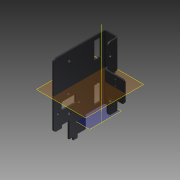
# Autodesk Inventor part: D-003
Saved by Autodesk Inventor 2015 (Build 190159000, 159)
## iProperties
Created: 2014-01-21
Part Number: D-003
Material: Steel
Document SubType Name: Chapa
Designer: O.Martin
Mass: 157.649 g
Surface Area: 219.047 cm^2
Volume: 20.0827 cm^3
Density: 7.85 g/cm^3
Project: WITBOXprinter_K01
Description: PLACA LATERAL MOTOR
Stock Number: 2014000004
Sheet Metal Rule: Por defecto
Appearance: Rubber - Black - Version 1.1
GlobalPropertyList: <PropertyList/>
Company: MARCHA TECHNOLOGY
Author: O.Martin
Autodesk Inventor part; units mm, degrees
ref_plane "YZ Plane" through (0, 0, 0) normal (1, 0, 0) x (0, 1, 0)
ref_plane "XZ Plane" through (0, 0, 0) normal (0, 1, 0) x (-1, 0, 0)
sketch "Boceto1" plane through (0, 0, 0) normal (0, 0, 1) x (1, 0, 0)
  line L0 (0, -25) -> (0, 25) construction
  circle A0 centre (0, 25) radius 4 construction
  circle A1 centre (0, 25) radius 7.5 construction
  line L1 (-7.5399, -37.5) -> (-7.5399, 37.5)
  line L2 (-7.5399, 37.5) -> (12.4601, 37.5)
  line L3 (12.4601, 37.5) -> (12.4601, 22)
  line L4 (12.4601, 22) -> (10.4601, 22)
  line L5 (10.4601, 22) -> (10.4601, 35.5)
  line L6 (10.4601, 35.5) -> (-5.5399, 35.5)
  line L7 (-5.5399, 35.5) -> (-5.5399, -35.5)
  line L8 (-5.5399, -35.5) -> (40.4601, -35.5)
  line L9 (40.4601, -35.5) -> (40.4601, -5)
  line L10 (40.4601, -5) -> (42.4601, -5)
  line L11 (42.4601, -5) -> (42.4601, -37.5)
  line L12 (42.4601, -37.5) -> (-7.5399, -37.5)
  line L13 (-5.5399, 19.9443) -> (-7.5399, 19.9443) construction
  line L14 (-5.5399, 30.0557) -> (-7.5399, 30.0557) construction
  line L15 (-5.5399, -35.5) -> (-5.5399, -37.5)
  point P0 (-7.5399, 0)
  point P1 (0, 0)
  point P2 (0, 0)
  dimension "d4" = 2
  dimension "d5" = 2
  dimension "d6" = 2
  dimension "d7" = 2
  dimension "d46" = 12.5
  dimension "d47" = 75
  dimension "d49" = 3
  dimension "d87" = 15
  dimension "d88" = 20
  dimension "d89" = 8
  dimension "d93" = 32.5
  dimension "d94" = 50
  dimension "d198" = 10.1114
  constraints: 32 end point, 12 parallel, 5 point on line, 4 perpendicular, 3 coincident, 2 centre point, 2 midpoint, 2 point on circle, 1 horizontal alignment, 1 vertical
  measures "d4" distance between parallel lines of L1 L7
  measures "d5" distance of L9.end L10.end
  measures "d6" distance between parallel lines of L12 L8
  measures "d7" distance between parallel lines of L2 L6
  measures "d46" distance from line of L2 L0.end
  measures "d47" distance between parallel lines of L12 L2
  measures "d49" distance from line of A0.centre L4
  measures "d87" diameter of A1
  measures "d88" distance of L1.end L2.end
  measures "d89" diameter of A0
  measures "d93" distance of L10.end L11.end
  measures "d94" distance of L11.end L1.start
  measures "d198" distance between parallel lines of L13 L14
extrude "Extrusión1" add sketch "Boceto1" along normal mid plane 90 contours L1 L2 L3 L4 L5 L6 L7 L15 L12
fillet "Empalme1" radius 4 6 edges at (-7.5399, 37.5, 0) (12.4601, 37.5, 0) (11.4601, 22, 45) (11.4601, 22, -45) (-6.5399, -37.5, 45) (-6.5399, -37.5, -45)
fillet "Empalme1" radius 2 2 edges at (-5.5399, 35.5, 0) (10.4601, 35.5, 0)
sketch "Boceto2" plane through (-7.5399, -33.5, 45) normal (-1, 0, 0) x (0, 0, 1)
  line L0 (-84.6, 63.3744) -> (-60.4, 63.3744)
  line L1 (-60.4, 63.3744) -> (-60.4, 53.6256)
  line L2 (-60.4, 53.6256) -> (-84.6, 53.6256)
  line L3 (-84.6, 53.6256) -> (-84.6, 63.3744)
  line L4 (-29.6, 53.6256) -> (-5.4, 53.6256)
  line L5 (-5.4, 53.6256) -> (-5.4, 63.3744)
  line L6 (-5.4, 63.3744) -> (-29.6, 63.3744)
  line L7 (-29.6, 63.3744) -> (-29.6, 53.6256)
  line L8 (-84.6, 18.5) -> (-5.4, 18.5) construction
  line L9 (-5.4, 18.5) -> (-5.4, 58.5) construction
  line L10 (-5.4, 58.5) -> (-84.6, 58.5) construction
  line L11 (-84.6, 58.5) -> (-84.6, 18.5) construction
  line L12 (0, 71) -> (-90, 71) projected
  line L13 (0, 0) -> (0, 67) projected
  line L14 (-72.5, 63.3744) -> (-72.5, 53.6256) construction
  line L15 (-90, 67) -> (0, 67) construction
  line L16 (-17.5, 63.3744) -> (-17.5, 53.6256) construction
  circle A0 centre (-60.4, 58.5) radius 1
  circle A1 centre (-29.6, 58.5) radius 1
  point P0 (-45, 18.5)
  point P1 (-12.5, 18.5)
  point P2 (-77.5, 18.5)
  point P3 (-72.5, 58.5)
  point P4 (-17.5, 58.5)
  point P5 (-45, 58.5)
  point P6 (-45, 67)
  dimension "d33" = 24.2
  dimension "d36" = 65
  dimension "d45" = 40
  dimension "d48" = 9.7488
  dimension "d103" = 12.5
  dimension "d165" = 12.5
  dimension "d186" = 55
  dimension "d286" = 2
  constraints: 28 end point, 11 midpoint, 8 parallel, 6 point on line, 5 perpendicular, 3 horizontal, 3 vertical alignment, 2 centre point, 1 equal radius
  measures "d33" distance of L4.start L4.end
  measures "d36" distance of point (-12.5, 18.5) point (-77.5, 18.5)
  measures "d45" distance between parallel lines of L10 L8
  measures "d48" distance of L4.end L5.end
  measures "d103" distance between parallel lines of L12 L10
  measures "d165" distance from line of L13 point (-12.5, 18.5)
  measures "d186" distance between parallel lines of L16 L14
  measures "d286" diameter of A0
extrude "Extrusión2" cut sketch "Boceto2" against normal blind 5
hole "Agujero2" at (-7.5399, -15, 32.5) at (-7.5399, -15, -32.5) direction (1, 0, 0) diameter 4 end through all
sketch "Boceto5" plane through (-7.5399, -33.5, 45) normal (-1, 0, 0) x (0, 0, 1)
  line L0 (-68.5, 27.2) -> (-57.5, 27.2)
  line L1 (-57.5, 27.2) -> (-57.5, 7.2)
  line L2 (-57.5, 7.2) -> (-68.5, 7.2)
  line L3 (-68.5, 7.2) -> (-68.5, 27.2)
  circle A0 centre (-77.5, 18.5) radius 2 projected
  line L4 (-90, 67) -> (-90, 0) projected
  line L5 (-69.5, 32.2) -> (-69.5, 2.2) construction
  point P0 (-63, 17.2)
  point P1 (-63, 27.2)
  point P2 (-68.5, 17.2)
  point P3 (-69.5, 17.2)
  dimension "d63" = 20
  dimension "d136" = 1.3
  dimension "d200" = 30
  dimension "d257" = 8
  dimension "d293" = 9
  dimension "d294" = 11
  constraints: 10 end point, 3 midpoint, 3 parallel, 2 horizontal alignment, 1 coincident, 1 horizontal, 1 perpendicular, 1 vertical alignment
  measures "d63" distance of L2.end L0.start
  measures "d136" vertical distance of point (-77.5, 18.5) point (-68.5, 17.2)
  measures "d200" distance of L5.start L5.end
  measures "d257" distance from line of A0.centre L5
  measures "d293" distance from line of L3 point (-77.5, 18.5)
  measures "d294" distance of L1.end L2.end
extrude "Extrusión4" cut sketch "Boceto5" against normal blind 3 contours L0 L1 L2 L3
fillet "Empalme3" radius 2 4 edges at (-6.5399, -6.3, -23.5) (-6.5399, -6.3, -12.5) (-6.5399, -26.3, -12.5) (-6.5399, -26.3, -23.5)
hole "Agujero5" at (-7.5399, 25, -27.5) at (-7.5399, 25, 27.5) direction (1, 0, 0) diameter 3.242 end through all thread size "M4x0.7" class "6H" standard "ISO Metric profile"
hole "Agujero6" at (-7.5399, -1.3, -24.5) at (-7.5399, -31.3, -24.5) direction (1, 0, 0) diameter 3.242 depth 8 tip angle 118 thread size "M4x0.7" class "6H" standard "ISO Metric profile"
sketch "Boceto7" plane through (-7.5399, -33.5, 45) normal (-1, 0, 0) x (0, 0, 1)
  circle A0 centre (-77.5, 18.5) radius 2 projected
  circle A1 centre (-12.5, 18.5) radius 2 projected
  line L0 (-90, 67) -> (-90, 0) projected
  line L1 (-12.5, 28.5) -> (-12.5, 8.5) construction
  line L2 (-77.5, 28.5) -> (-77.5, 8.5) construction
  dimension "d113" = 20
  constraints: 6 coincident, 4 end point, 3 parallel, 2 midpoint
  measures "d113" distance of L1.start L1.end
hole "Agujero8" [suppressed]
sketch "Boceto8" plane through (-3.5399, 37.5, -45) normal (0, 1, 0) x (1, 0, 0)
  line L0 (0, -90) -> (12, -90) projected
  line L1 (4.2, -20) -> (4.2, -70) construction
  line L2 (-4, 0) -> (-4, -90) construction
  point P0 (4.2, -45)
  dimension "d121" = 8.2
  dimension "d122" = 50
  dimension "d169" = 20
  constraints: 2 coincident, 2 end point, 1 midpoint, 1 perpendicular
  measures "d121" distance between parallel lines of L2 L1
  measures "d122" distance of L1.start L1.end
  measures "d169" distance from line of L0 point (4.2, -70)
hole "Agujero9" [suppressed]
sketch "Boceto10" plane through (-7.5399, -33.5, 45) normal (-1, 0, 0) x (0, 0, 1)
  line L0 (-4, -4) -> (-86, -4) projected
  line L1 (-90, 67) -> (-90, 0) projected
  line L2 (-90, 18) -> (-86, 18)
  line L3 (-86, 18) -> (-86, 8)
  line L4 (-86, 8) -> (-90, 8)
  line L5 (-90, 8) -> (-90, 18)
  dimension "d137" = 4
  dimension "d139" = 10
  dimension "d195" = 22
  constraints: 8 end point, 2 parallel, 1 horizontal, 1 perpendicular, 1 point on line
  measures "d137" distance between parallel lines of L1 L3
  measures "d139" distance of L2.end L3.end
  measures "d195" distance between parallel lines of L2 L0
extrude "Extrusión6" cut sketch "Boceto10" against normal through all
sketch "Boceto14" plane through (0, 0, 0) normal (0, 0, 1) x (1, 0, 0)
  line L0 (10.4601, 22) -> (12.4601, 22) projected
  line L1 (12.4601, 22) -> (12.4601, 21)
  arc A0 (12.4601, 21) -> (14.4601, 19) centre (14.4601, 21) ccw
  line L2 (14.4601, 19) -> (40.4601, 19)
  line L3 (40.4601, 19) -> (40.4601, 17)
  line L4 (40.4601, 17) -> (14.4601, 17)
  arc A1 (10.4601, 21) -> (14.4601, 17) centre (14.4601, 21) ccw
  line L5 (10.4601, 21) -> (10.4601, 22)
  dimension "d161" = 4
  dimension "d189" = 5
  dimension "d190" = 30
  constraints: 10 end point, 4 point on circle, 4 tangent, 3 parallel, 2 centre point, 2 perpendicular, 1 concentric
  measures "d161" radius of A1
  measures "d189" distance between parallel lines of L0 L4
  measures "d190" distance between parallel lines of L5 L3
extrude "Extrusión8" add sketch "Boceto14" along normal mid plane 30
sketch "Boceto15" plane through (14.4601, 19, 15) normal (0, 1, 0) x (1, 0, 0)
  line L0 (0, 0) -> (26, 0) projected
  line L1 (26, 0) -> (26, 30) projected
  line L2 (0, 0) -> (0, 30) projected
  line L3 (13, 4.5) -> (13, 12.5) construction
  dimension "d170" = 13
  dimension "d171" = 4.5
  dimension "d172" = 8
  constraints: 2 coincident, 2 end point, 1 parallel
  measures "d170" distance between parallel lines of L1 L3
  measures "d171" distance from line of L0 L3.start
  measures "d172" distance of L3.start L3.end
hole "Agujero11" at (27.4601, 19, 10.5) at (27.4601, 19, 2.5) direction (0, -1, 0) diameter 2.459 end through all thread size "M3x0.5" class "6H" standard "ISO Metric profile"
fillet "Empalme4" radius 4 2 edges at (40.4601, 18, 15) (40.4601, 18, -15)
feature "Desplazar cara1" [suppressed]
sketch "Boceto18" plane through (-3.5399, 37.5, -45) normal (0, 1, 0) x (1, 0, 0)
  line L0 (0, -90) -> (0, 0) projected
  line L1 (16, -90) -> (16, 0) projected
  line L2 (16, -42.25) -> (2, -42.25)
  line L3 (2, -42.25) -> (2, -39.75)
  line L4 (2, -39.75) -> (16, -39.75)
  line L5 (16, -39.75) -> (16, -42.25)
  line L6 (16, -47.75) -> (2, -47.75)
  line L7 (2, -47.75) -> (2, -50.25)
  line L8 (2, -50.25) -> (16, -50.25)
  line L9 (16, -50.25) -> (16, -47.75)
  line L10 (2, -42.25) -> (2, -47.75) construction
  line L11 (12, 0) -> (12, -90) projected
  line L12 (16, -42.25) -> (16, -47.75)
  line L13 (11, -42.25) -> (11, -47.75)
  point P0 (2, -45)
  point P1 (0, -45)
  dimension "d202" = 5.5
  dimension "d203" = 2.5
  dimension "d207" = 1
  dimension "d208" = 9
  constraints: 22 end point, 5 parallel, 4 point on line, 3 perpendicular, 2 equal length, 2 horizontal, 2 midpoint, 1 collinear, 1 horizontal alignment
  measures "d202" distance between parallel lines of L6 L2
  measures "d203" distance of L2.end L3.end
  measures "d207" distance between parallel lines of L11 L13
  measures "d208" distance between parallel lines of L3 L13
extrude "Extrusión11" cut sketch "Boceto18" against normal blind 8
fillet "Redondeo de esquina1" radius 1.25 8 edges at (-1.5399, 36.5, -5.25) (-1.5399, 36.5, -2.75) (-1.5399, 36.5, 2.75) (-1.5399, 36.5, 5.25) (7.4601, 36.5, 2.75) (7.4601, 36.5, -2.75) (11.4601, 29.5, -5.25) (11.4601, 29.5, 5.25)
sketch "Boceto21" plane through (12.4601, 26, 45) normal (1, 0, 0) x (0, 0, -1)
  line L0 (49, 3.5) -> (41, 3.5) projected
  line L1 (39.75, 11.5) -> (0, 11.5) projected
  point P0 (45, -1)
  point P1 (45, 3.5)
  dimension "d224" = 12.5
  constraints: 1 midpoint, 1 vertical alignment
  measures "d224" distance from line of point (45, -1) L1
hole "Agujero12" [suppressed]
sketch "Boceto22" plane through (-7.5399, -33.5, 45) normal (-1, 0, 0) x (0, 0, 1)
  line L0 (-90, 67) -> (-90, 0)
  line L1 (-90, 18) -> (-109, 18)
  line L2 (-109, 18) -> (-109, 24)
  line L3 (-109, 24) -> (-113, 24)
  line L4 (-113, 24) -> (-113, 30)
  line L5 (-113, 30) -> (-90, 30)
  line L6 (-90, 67) -> (-90, 18) projected
  dimension "d232" = 12
  dimension "d233" = 6
  dimension "d234" = 19
  dimension "d235" = 4
  constraints: 12 end point, 2 parallel, 2 perpendicular, 2 point on line
  measures "d232" distance between parallel lines of L1 L5
  measures "d233" distance of L3.end L4.end
  measures "d234" distance of L1.start L1.end
  measures "d235" distance of L2.end L3.end
extrude "Extrusión13" add sketch "Boceto22" against normal up to surface (2 mm away)
ref_plane "Plano de trabajo1" through (0, 0, -47) normal (0, 0, -1) x (-1, 0, 0)
sketch "Boceto23" plane through (0, 0, -47) normal (0, 0, -1) x (-1, 0, 0)
  line L0 (5.5399, -3.5) -> (7.5399, -3.5) projected
  line L1 (7.5399, -3.5) -> (7.5399, 6.5)
  arc A0 (9.3655, 8.4924) -> (7.5399, 6.5) centre (9.5399, 6.5) ccw
  line L2 (9.3655, 8.4924) -> (23.3123, 9.7126)
  line L3 (23.3123, 9.7126) -> (23.138, 11.705)
  line L4 (23.138, 11.705) -> (9.1912, 10.4848)
  arc A1 (9.1912, 10.4848) -> (5.5399, 6.5) centre (9.5399, 6.5) ccw
  line L5 (5.5399, -3.5) -> (5.5399, 6.5)
  line L6 (9.3655, 8.4924) -> (306.3655, 8.4924) construction
  line L7 (23.3123, 9.7126) -> (306.3655, 34.4765) construction
  line L8 (306.3655, 8.4924) -> (306.3655, 34.4765) construction
  dimension "d239" = 2
  dimension "d287" = 10
  dimension "d288" = 14
  dimension "d289" = 95
  dimension "d290" = 2
  dimension "d291" = 297
  dimension "d292" = 25.9841
  constraints: 16 end point, 4 perpendicular, 4 point on circle, 4 tangent, 2 centre point, 2 parallel, 1 concentric
  measures "d239" radius of A0
  measures "d287" distance from line of A0.centre L0
  measures "d288" distance of L3.end L4.end
  measures "d289" angle of L5 L4
  measures "d290" radial gap between concentric circles of A0 A1
  measures "d291" distance of L2.start L6.end
  measures "d292" distance of L6.end L7.end
extrude "Extrusión14" add sketch "Boceto23" along normal blind 16
sketch "Boceto24" plane through (-5.5399, -33.5, 45) normal (1, 0, 0) x (0, 0, -1)
  line L0 (92, 40) -> (108, 40) projected
  line L1 (92, 40) -> (92, 30) projected
  line L2 (90, 30) -> (92, 30) projected
  line L3 (90, 30) -> (90, 67) projected
  line L4 (90, 38) -> (92, 38) construction
  arc A0 (90, 38) -> (92, 38) centre (91, 38) ccw
  point P0 (109, 41)
  dimension "d244" = 2
  constraints: 2 end point, 2 point on circle, 2 point on line, 1 centre point, 1 midpoint, 1 perpendicular, 1 other
  measures "d244" length of L4
extrude "Extrusión15" add sketch "Boceto24" against normal up to surface (2 mm away)
sketch "Boceto25" plane through (-23.138, 11.705, -47) normal (0.0871557, 0.9961947, 0) x (0.9961947, -0.0871557, 0)
  line L0 (0, 0) -> (0, 16) projected
  line L1 (14, 0) -> (14, 16) projected
  line L2 (12, 8) -> (4, 8) construction
  point P0 (0, 8)
  dimension "d247" = 4
  dimension "d248" = 8
  constraints: 2 coincident, 2 end point, 1 horizontal alignment, 1 midpoint, 1 perpendicular
  measures "d247" distance from line of L0 L2.end
  measures "d248" distance of L2.start L2.end
hole "Agujero13" at (-11.1836, 10.6591, -55) at (-19.1532, 11.3563, -55) direction (-0.0871557, -0.9961947, 0) diameter 2.459 depth 2 tip angle 118 thread size "M3x0.5" class "6H" standard "ISO Metric profile"
fillet "Empalme6" radius 2 2 edges at (-23.2251, 10.7088, -63) (-23.2251, 10.7088, -47)
sketch "Boceto26" plane through (-7.5399, -33.5, 45) normal (-1, 0, 0) x (0, 0, 1)
  circle A0 centre (-69.5, 32.2) radius 1.621 projected
  line L0 (-57.5, 25.2) -> (-57.5, 9.2) projected
  point P0 (-52, 17.2)
  point P1 (-57.5, 17.2)
  dimension "d259" = 17.5
  constraints: 1 horizontal alignment, 1 midpoint
  measures "d259" horizontal distance of point (-52, 17.2) A0.centre
hole "Agujero14" at (-7.5399, -16.3, -7) direction (1, 0, 0) diameter 3.242 depth 8 tip angle 118 thread size "M4x0.7" class "6H" standard "ISO Metric profile"
sketch "Boceto27" plane through (-3.5399, 37.5, -45) normal (0, 1, 0) x (1, 0, 0)
  line L0 (11, -46.5) -> (11, -43.5) projected
  point P0 (7, -45)
  point P1 (11, -45)
  dimension "d267" = 4
  constraints: 1 horizontal alignment, 1 midpoint
  measures "d267" distance from line of point (7, -45) L0
hole "Agujero15" [suppressed]
sketch "Boceto28" plane through (-3.5399, 37.5, -45) normal (0, 1, 0) x (1, 0, 0)
  line L0 (12, 0) -> (0, 0) projected
  line L1 (3.25, -47.75) -> (9.75, -47.75) projected
  line L2 (5.5, -4) -> (5.5, -22) construction
  line L3 (-2, -90) -> (-2, 0) construction
  line L4 (-4, 0) -> (-4, -90) projected
  dimension "d275" = 18
  dimension "d277" = 4
  dimension "d285" = 9.5
  constraints: 2 coincident, 2 end point, 1 perpendicular
  measures "d275" distance of L2.start L2.end
  measures "d277" distance from line of L0 L2.start
  measures "d285" distance between parallel lines of L4 L2
hole "Agujero16" [suppressed]
sketch "Boceto20" plane through (12.4601, 26, 45) normal (1, 0, 0) x (0, 0, -1)
  line L0 (0, 7.5) -> (0, 0) projected
  arc A0 (0, 0) -> (4, -4) centre (4, 0) ccw projected
  line L1 (30, -4) -> (4, -4) projected
  line L2 (39.75, 11.5) -> (0, 11.5) projected
  line L3 (22, 7.5) -> (22, 11.5)
  arc A1 (21, 6.5) -> (22, 7.5) centre (21, 7.5) ccw
  line L4 (0, 11.5) -> (0, 7.5)
  line L5 (49, 3.5) -> (41, 3.5) projected
  line L6 (15, -1) -> (15, 5.5)
  arc A2 (16, 6.5) -> (15, 5.5) centre (16, 5.5) ccw
  line L7 (16, 6.5) -> (21, 6.5)
  arc A3 (15, -1) -> (18, -4) centre (18, -1) ccw
  line L8 (0, 7.5) -> (39.75, 7.5) projected
  line L9 (16, 6.5) -> (1, 6.5)
  arc A4 (1, 6.5) -> (0, 5.5) centre (1, 5.5) ccw
  dimension "d212" = 22
  dimension "d216" = 1
  dimension "d221" = 5
  dimension "d222" = 15
  dimension "d223" = 3
  constraints: 10 end point, 9 tangent, 8 point on circle, 4 centre point, 3 point on line, 2 equal radius, 2 parallel, 2 perpendicular
  measures "d212" distance from line of L2.end L3
  measures "d216" radius of A1
  measures "d221" distance between parallel lines of L2 L7
  measures "d222" distance between parallel lines of L0 L6
  measures "d223" radius of A3
equation "\"d5\" = d4"
equation "\"d6\" = d4"
equation "\"d7\" = d4"
equation "\"d48\" = d12"
equation "\"d12\" = 9.748846"
body "Solid1"
